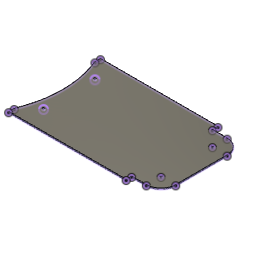
magnetic catch bag v1 (Autodesk Fusion 360 design; units mm, degrees)
Autodesk Fusion 360 part; units mm, degrees
sketch "Sketch1" plane through (0, 0, 0) normal (0, 1, 0) x (1, 0, 0)
  line L0 (80, -125) -> (-80, -125)
  line L1 (-80, -125) -> (-80, 125)
  line L2 (-80, 125) -> (80, 125)
  line L3 (80, 125) -> (80, -125)
  line L4 (80, -125) -> (-80, 125) construction
  line L5 (-80, -125) -> (80, 125) construction
  line L6 (80, 125) -> (240, 125)
  line L7 (240, 125) -> (240, -125)
  line L8 (240, -125) -> (80, -125)
  line L9 (80, -125) -> (80, 125)
  line L10 (240, 110) -> (280, 110)
  line L11 (2.5, 0) -> (20, 0)
  line L12 (240, -110) -> (280, -110)
  line L13 (320, 70) -> (320, -70)
  arc A0 (-80, -110) -> (-80, 110) centre (-344, 0) ccw
  line L14 (0, 0) -> (-80, 0) construction
  arc A1 (320, 70) -> (280, 110) centre (280, 70) ccw
  arc A2 (280, -110) -> (320, -70) centre (280, -70) ccw
  line L15 (280, 70) -> (-271.7196, 70) construction
  line L16 (280, -70) -> (-262.1178, -70) construction
  circle A3 centre (280, 70) radius 2.5
  circle A4 centre (280, -70) radius 2.5
  circle A5 centre (-40, 70) radius 2.5
  circle A6 centre (-40, -70) radius 2.5
  point P0 (320, 110)
  point P1 (-80, 110)
  point P2 (-80, -110)
  point P3 (-58, 0)
  dimension "d1" = 160
  dimension "d2" = 250
  dimension "d3" = 160
  dimension "d4" = 80
  dimension "d5" = 15
  dimension "d6" = 15
  dimension "d7" = 15
  dimension "d8" = 22
  dimension "d9" = 40
  dimension "d10" = 5
  dimension "d11" = 5
  dimension "d12" = 5
  dimension "d13" = 5
  dimension "d14" = 40
  dimension "d15" = 40
  constraint horizontal L0
  constraint perpendicular L0 L1
  constraint parallel L0 L2
  constraint parallel L1 L3
  constraint coincident L4 L14.start
  constraint coincident L5 L14.start
  constraint coincident L14.start origin
  constraint horizontal L6
  constraint vertical L7
  constraint horizontal L8
  constraint vertical L9
  constraint collinear L0 L8
  constraint coincident L7 L10.start
  constraint perpendicular L7 L10
  constraint symmetric L10.start L11 L12.start
  constraint coincident L1 P1
  constraint coincident L1 P2
  constraint coincident P2 A0.start
  constraint coincident P1 A0.end
  constraint midpoint L1 L14.end
  constraint midpoint A0 P3
  constraint coincident P0 L10
  constraint coincident P0 L13
  constraint tangent L10 A1
  constraint tangent L13 A1
  constraint tangent L13 A2
  constraint tangent L12 A2
  constraint equal A1 A2
  constraint coincident A1.centre L15.start
  constraint perpendicular L7 L15
  constraint coincident A2.centre L16.start
  constraint horizontal L16
  constraint concentric A1 A3
  constraint concentric A2 A4
  constraint coincident L15 A5.centre
  constraint coincident L16 A6.centre
  measures "d1" distance of L1.end L2.end
  measures "d2" distance of L0.end L1.end
  measures "d3" distance of L2.end L6.end
  measures "d4" distance of L10.start P0
  measures "d5" distance of L6 L10
  measures "d6" distance of L2 P1
  measures "d7" distance of L0 P2
  measures "d8" distance of L1 P3
  measures "d9" radius of A1
  measures "d10" diameter of A3
  measures "d11" diameter of A4
  measures "d12" diameter of A5
  measures "d13" diameter of A6
  measures "d14" distance of L1 A5.centre
  measures "d15" distance of L1 A6.centre
extrude "Extrude1" add sketch "Sketch1" along normal blind 3 contours L0 L1 L2 L3 L9 A0 | L3 L6 L7 L8 L9 | L7 L10 L12 L13 A1 A2
sketch "Sketch2" plane through (0, 0, 0) normal (0, 1, 0) x (1, 0, 0)
  circle A0 centre (280, 70) radius 2.5
  circle A1 centre (-40, -70) radius 2.5
  circle A2 centre (-40, 70) radius 2.5
  circle A3 centre (280, -70) radius 2.5
  line L0 (240, -110) -> (280, -110)
  arc A4 (280, -110) -> (320, -70) centre (280, -70) ccw
  line L1 (320, -70) -> (320, 70)
  arc A5 (320, 70) -> (280, 110) centre (280, 70) ccw
  line L2 (280, 110) -> (240, 110)
  line L3 (240, 110) -> (240, 125)
  line L4 (240, 125) -> (-80, 125)
  line L5 (-80, 125) -> (-80, 110)
  arc A6 (-80, -110) -> (-80, 110) centre (-344, 0) ccw
  line L6 (-80, -110) -> (-80, -125)
  line L7 (-80, -125) -> (240, -125)
  line L8 (240, -125) -> (240, -110)
